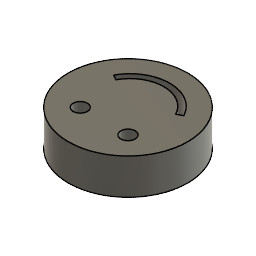
_Animation Test Print.c652fa5c-e650-4809-80f6-2eb2ca7b7716 (Autodesk Fusion 360 design; units mm, degrees)
Autodesk Fusion 360 part; units mm, degrees
sketch "Sketch1" plane through (0, 0, 0) normal (0, 1, 0) x (1, 0, 0)
  line L0 (-25, 13.3333) -> (-29.4118, 15.6863)
  line L1 (25, 13.3333) -> (29.4118, 15.6863)
  circle A0 centre (20, -21.6667) radius 6
  arc A1 (29.4118, 15.6863) -> (-29.4118, 15.6863) centre (0, 0) ccw
  circle A2 centre (-20, -21.6667) radius 6
  arc A3 (25, 13.3333) -> (-25, 13.3333) centre (0, 0) ccw
  circle A4 centre (0, -1.6667) radius 50
  line L2 (0, -1.6667) -> (0, -26.6667)
  dimension "d1" = 5
  dimension "d2" = 100
  dimension "d3" = 12
  constraint coincident A4.centre L2.start
  constraint vertical L2
  constraint symmetric A0 A2 L2
  measures "d2" diameter of A4
  measures "d3" diameter of A0
extrude "Extrude1" add sketch "Sketch1" along normal blind 30
